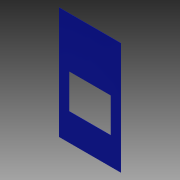
# Autodesk Inventor part: GE-13012R
Saved by Autodesk Inventor 2013 (Build 170138000, 138)
## iProperties
Created: 2013-01-03
Part Number: GE-13012R
Material: Polyethylene, High Density
Document SubType Name: Modeling
Designer: Phillip
Density: 1 g/cm^3
Author: Phillip
Autodesk Inventor part; units mm, degrees
ref_plane "YZ Plane" through (0, 0, 0) normal (1, 0, 0) x (0, 1, 0)
ref_plane "XZ Plane" through (0, 0, 0) normal (0, 1, 0) x (-1, 0, 0)
ref_plane "XY Plane" through (0, 0, 0) normal (0, 0, 1) x (1, 0, 0)
sketch "Sketch1" plane through (0, 0, 0) normal (0, 0, 1) x (1, 0, 0)
  line L0 (-546.1, -990.6) -> (546.1, -990.6)
  line L1 (546.1, -990.6) -> (546.1, 990.6)
  line L2 (546.1, 990.6) -> (-546.1, 990.6)
  line L3 (-546.1, 990.6) -> (-546.1, -990.6)
  line L4 (-546.1, -990.6) -> (546.1, 990.6) construction
  line L5 (546.1, -990.6) -> (-546.1, 990.6) construction
  point P0 (0, 0)
  dimension "d0" = 1092.2
  dimension "d1" = 1981.2
  constraints: 12 end point, 2 midpoint, 2 parallel, 1 horizontal, 1 perpendicular
  measures "d0" distance of L2.end L1.end
  measures "d1" distance of L1.end L0.end
extrude "Extrusion1" add sketch "Sketch1" against normal blind 3.175
sketch "Sketch2" plane through (0, 0, 0) normal (0, 0, 1) x (1, 0, 0)
  line L0 (546.1, 990.6) -> (-546.1, 990.6) projected
  line L1 (-546.1, 990.6) -> (-546.1, -990.6) projected
  line L2 (-368.3, -508) -> (368.3, -508)
  line L3 (368.3, -508) -> (368.3, 101.6)
  line L4 (368.3, 101.6) -> (-368.3, 101.6)
  line L5 (-368.3, 101.6) -> (-368.3, -508)
  point P0 (0, 0)
  dimension "d4" = 736.6
  dimension "d6" = 609.6
  dimension "d7" = 889
  dimension "d8" = 177.8
  constraints: 8 end point, 2 parallel, 1 horizontal, 1 perpendicular
  measures "d4" distance of L3.end L4.end
  measures "d6" distance of L2.end L3.end
  measures "d7" distance between parallel lines of L4 L0
  measures "d8" distance between parallel lines of L5 L1
extrude "Extrusion2" cut sketch "Sketch2" against normal up to next
body "Solid1"
